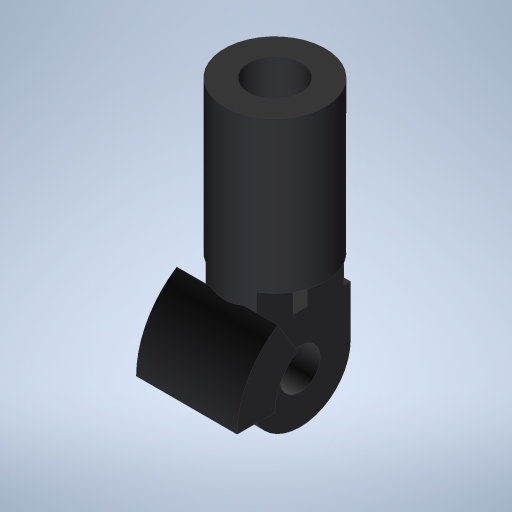
# Autodesk Inventor part: hingejoint1
Saved by Autodesk Inventor 2024 (Build 280153000, 153)
## iProperties
Created: 2024-05-16
Part Number: hingejoint1
Material: Generic
Document SubType Name: Modeling
Designer: maja6
Density: 1 g/cm^3
Appearance: Default
Author: maja6
Autodesk Inventor part; units mm, degrees
ref_plane "YZ Plane" through (0, 0, 0) normal (1, 0, 0) x (0, 1, 0)
ref_plane "XZ Plane" through (0, 0, 0) normal (0, 1, 0) x (-1, 0, 0)
ref_plane "XY Plane" through (0, 0, 0) normal (0, 0, 1) x (1, 0, 0)
sketch "Sketch1" plane through (0, 0, 0) normal (0, 0, 1) x (1, 0, 0)
  circle A0 centre (0, 0) radius 2
  circle A1 centre (0, 0) radius 4
  dimension "d0" = 4
  dimension "d1" = 8
  constraints: 2 centre point, 2 coincident
  measures "d0" diameter of A0
  measures "d1" diameter of A1
extrude "Extrusion1" add sketch "Sketch1" along normal blind 15
sketch "Sketch2" plane through (0, 0, 0) normal (0, 0, -1) x (-1, 0, 0)
  circle A0 centre (0, 0) radius 4 projected
  line L0 (0, 4) -> (4, 4)
  line L1 (4, 4) -> (4, -4)
  line L2 (4, -4) -> (0, -4)
  line L3 (0, -4) -> (0, 4)
  line L4 (4, -4) -> (-4, -4)
  line L5 (-4, -4) -> (-4, 4)
  line L6 (-4, 4) -> (4, 4)
  line L7 (4, 4) -> (4, -4)
  constraints: 16 end point, 4 parallel, 2 horizontal, 2 perpendicular, 1 point on line, 1 vertical alignment, 1 other
extrude "Extrusion2" add sketch "Sketch2" along normal blind 8
sketch "Sketch3" plane through (4, 0, 0) normal (1, 0, 0) x (0, 0, -1)
  circle A0 centre (4, 0) radius 4
  line L0 (0, 4) -> (0, 0) projected
  line L1 (8, 4) -> (8, -4) projected
  line L2 (0, 4) -> (8, 4)
  line L3 (8, 4) -> (8, -4)
  line L4 (8, -4) -> (0, -4)
  line L5 (0, -4) -> (0, 4)
  point P0 (4, -4)
  point P1 (8, 0)
  point P2 (4, 4)
  constraints: 8 end point, 2 parallel, 1 centre point, 1 horizontal, 1 perpendicular
extrude "Extrusion3" cut sketch "Sketch3" against normal blind 8 contours L1 L4 A0 | A0 L2 L1
sketch "Sketch4" plane through (4, 0, 0) normal (1, 0, 0) x (0, 0, -1)
  circle A0 centre (4.0004, 0) radius 1.6
  point P0 (0, 0)
  dimension "d8" = 3.2
  constraints: 1 centre point
  measures "d8" diameter of A0
extrude "Extrusion4" cut sketch "Sketch4" against normal blind 8
sketch "Sketch5" plane through (0, 0, 0) normal (0, 0, 1) x (1, 0, 0)
  line L0 (0, 4) -> (4, 4) projected
  line L1 (0, -4) -> (-4, -4) projected
  line L2 (2, 4) -> (-2, 4)
  line L3 (-2, 4) -> (-2, -4)
  line L4 (-2, -4) -> (2, -4)
  line L5 (2, -4) -> (2, 4)
  line L6 (4, -4) -> (0, -4) projected
  line L7 (4, -4) -> (-4, -4)
  line L8 (-4, -4) -> (-4, 4)
  line L9 (-4, 4) -> (4, 4)
  line L10 (4, 4) -> (4, -4)
  point P0 (0, 0)
  constraints: 16 end point, 4 parallel, 2 horizontal, 2 midpoint, 2 perpendicular
extrude "Extrusion5" cut sketch "Sketch5" against normal blind 8 contours L0 L10 L6 L5 | L3 L1 L8 L9
sketch "Sketch6" plane through (0, -4, 0) normal (0, -1, 0) x (1, 0, 0)
  line L0 (-2, -4) -> (2, -4) projected
  line L1 (-2, 0) -> (-4, 0) projected
  line L2 (0, -4) -> (-4, -4)
  line L3 (-4, -4) -> (-4, 0)
  line L4 (-4, 0) -> (0, 0)
  line L5 (0, 0) -> (0, -4)
  line L6 (0, -4) -> (3.9704, -4)
  line L7 (3.9704, -4) -> (3.9704, 0)
  line L8 (3.9704, 0) -> (0, 0)
  line L9 (0, 0) -> (0, -4)
  constraints: 16 end point, 4 parallel, 2 horizontal, 2 perpendicular, 1 midpoint, 1 point on line
extrude "Extrusion6" add sketch "Sketch6" along normal blind 3
sketch "Sketch7" plane through (0, 0, 0) normal (0, 0, -1) x (-1, 0, 0)
  line L0 (2, 4) -> (-2, 4) projected
  line L1 (-2, -4) -> (-2, 4) projected
  line L2 (2, 4) -> (-2, 4)
  line L3 (-2, 4) -> (-2, -4)
  line L4 (-2, -4) -> (2, -4)
  line L5 (2, -4) -> (2, 4)
  line L6 (5.0463, 4) -> (-4.8372, 4)
  line L7 (-4.8372, 4) -> (-4.8372, -4)
  line L8 (-4.8372, -4) -> (5.0463, -4)
  line L9 (5.0463, -4) -> (5.0463, 4)
  point P0 (0, 0)
  constraints: 16 end point, 4 parallel, 2 horizontal, 2 perpendicular, 2 point on line
extrude "Extrusion7" cut sketch "Sketch7" against normal blind 3 contours L6 L9 L8 L5 | L1 L8 L7 L6
sketch "Sketch8" plane through (-2, 3.4641, 0) normal (-1, 0, 0) x (0, 0, 1)
  circle A0 centre (-3.9998, -3.4641) radius 4
  circle A1 centre (-3.9998, -3.4641) radius 6.9959
  line L0 (-0.6612, -5.6672) -> (1.8871, -7.244)
  line L1 (-3.9998, -7.4641) -> (-3.9998, -10.46)
  circle A2 centre (-3.9998, -3.4641) radius 8.7454
  line L2 (0.613, -8.7238) -> (1.7591, -10.0457)
  line L3 (-5.354, -10.3276) -> (-5.7862, -12.0251)
  point P0 (0, -3.4641)
  constraints: 8 end point, 8 point on circle, 3 centre point, 2 coincident, 1 vertical
extrude "Extrusion8" cut sketch "Sketch8" along normal mid plane 20 contours A1 L2 A2 L3 picked at (0.8234, -9.9865)
extrude "Extrusion9" add sketch "Sketch8" along normal blind 2 and the other way blind 6 contours A0 L0 A1 L1 picked at (-3.4455, -9.3945)
sketch "Sketch9" plane through (0, 0, 15) normal (0, 0, 1) x (1, 0, 0)
  arc A0 (2, 0) -> (-2, 0) centre (0, 0) ccw projected
  circle A1 centre (0, 0) radius 2.075
  dimension "d23" = 4.15
  constraints: 1 centre point, 1 coincident
  measures "d23" diameter of A1
extrude "Extrusion10" cut sketch "Sketch9" against normal blind 15
body "Solid1"
